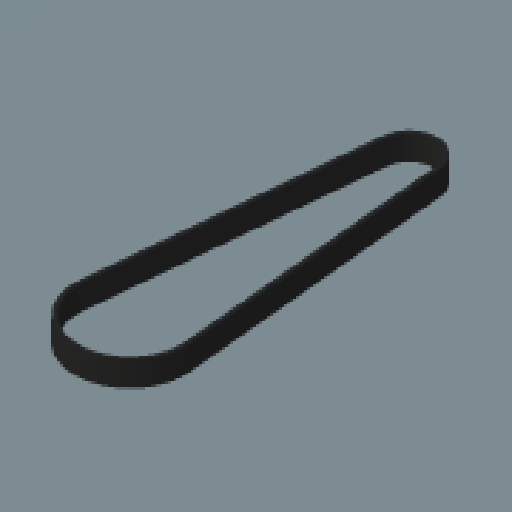
# Autodesk Inventor part: Z Axis Belt
Saved by Autodesk Inventor 2023.2 (Build 272271000, 271)
## iProperties
Created: 2023-02-15
Part Number: Z Axis Belt
Material: Rubber
Document SubType Name: Modeling
Designer: remop
Density: 0.93 g/cm^3
Appearance: Rubber - Black
Author: remop
Autodesk Inventor part; units mm, degrees
ref_plane "YZ Plane" through (0, 0, 0) normal (1, 0, 0) x (0, 1, 0)
ref_plane "XZ Plane" through (0, 0, 0) normal (0, 1, 0) x (-1, 0, 0)
ref_plane "XY Plane" through (0, 0, 0) normal (0, 0, 1) x (1, 0, 0)
sketch "Sketch1" plane through (0, 0, 0) normal (0, 1, 0) x (-1, 0, 0)
  line L0 (0, -23.2452) -> (0, 23.2452) construction
  line L1 (0, -34) -> (0, 34) construction
  arc A0 (12.4428, 32.8051) -> (-12.4428, 32.8051) centre (0, 34) ccw
  arc A1 (-5.9725, -34.5735) -> (5.9725, -34.5735) centre (0, -34) ccw
  line L2 (-12.4428, 32.8051) -> (-5.9725, -34.5735)
  line L3 (5.9725, -34.5735) -> (12.4428, 32.8051)
  arc A2 (13.4382, 32.7096) -> (-13.4382, 32.7096) centre (0, 34) ccw
  line L4 (13.4382, 32.7096) -> (6.9679, -34.6691)
  arc A3 (-6.9679, -34.6691) -> (6.9679, -34.6691) centre (0, -34) ccw
  line L5 (-6.9679, -34.6691) -> (-13.4382, 32.7096)
  point P0 (0, 0)
  dimension "d5" = 25
  dimension "d6" = 12
  dimension "d7" = 68
  dimension "d8" = 1
  constraints: 16 end point, 8 point on circle, 4 centre point, 4 tangent, 2 coincident, 2 midpoint, 1 point on line, 1 vertical, 3 other
  measures "d5" diameter of A0
  measures "d6" diameter of A1
  measures "d7" distance of L1.start L1.end
  measures "d8" radial gap between concentric circles of A2 A0
extrude "Extrusion1" add sketch "Sketch1" along normal blind 6
body "Solid1"
